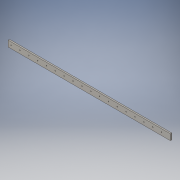
# Autodesk Inventor part: RailBar
Saved by Autodesk Inventor 2016 (Build 200138000, 138)
## iProperties
Created: 2015-08-23
Part Number: RailBar
Material: Stainless Steel
Document SubType Name: Modeling
Designer: myhome
Mass: 3520 g
Surface Area: 1108 cm^2
Volume: 440 cm^3
Density: 8 g/cm^3
Appearance: Semi-Polished
Author: myhome
Autodesk Inventor part; units mm, degrees
ref_plane "YZ Plane" through (0, 0, 0) normal (1, 0, 0) x (0, 1, 0)
ref_plane "XZ Plane" through (0, 0, 0) normal (0, 1, 0) x (-1, 0, 0)
ref_plane "XY Plane" through (0, 0, 0) normal (0, 0, 1) x (1, 0, 0)
sketch "Sketch1" plane through (0, 0, 0) normal (0, 0, 1) x (1, 0, 0)
  line L0 (0, 0) -> (1100, 0)
  line L1 (1100, 0) -> (1100, 40)
  line L2 (1100, 40) -> (0, 40)
  line L3 (0, 40) -> (0, 0)
  line L4 (1100, 40) -> (1040, 40)
  line L5 (1040, 40) -> (980, 40)
  line L6 (980, 40) -> (920, 40)
  line L7 (920, 40) -> (860, 40)
  line L8 (860, 40) -> (800, 40)
  line L9 (800, 40) -> (740, 40)
  line L10 (740, 40) -> (680, 40)
  line L11 (680, 40) -> (620, 40)
  line L12 (620, 40) -> (560, 40)
  line L13 (560, 40) -> (500, 40)
  line L14 (500, 40) -> (440, 40)
  line L15 (440, 40) -> (380, 40)
  line L16 (380, 40) -> (320, 40)
  line L17 (320, 40) -> (260, 40)
  line L18 (260, 40) -> (200, 40)
  line L19 (200, 40) -> (140, 40)
  line L20 (140, 40) -> (80, 40)
  line L21 (80, 40) -> (20, 40)
  circle A0 centre (1040, 20) radius 3
  circle A1 centre (980, 20) radius 3
  circle A2 centre (920, 20) radius 3
  circle A3 centre (860, 23) radius 3
  circle A4 centre (800, 20) radius 3
  circle A5 centre (740, 20) radius 3
  circle A6 centre (680, 20) radius 3
  circle A7 centre (560, 20) radius 3
  circle A8 centre (500, 20) radius 3
  circle A9 centre (440, 20) radius 3
  circle A10 centre (380, 20) radius 3
  circle A11 centre (320, 20) radius 3
  circle A12 centre (260, 20) radius 3
  circle A13 centre (200, 20) radius 3
  circle A14 centre (140, 20) radius 3
  circle A15 centre (80, 20) radius 3
  circle A16 centre (20, 20) radius 3
  dimension "d0" = 1100
  dimension "d1" = 40
  dimension "d22" = 6
  dimension "d23" = 6
  dimension "d24" = 6
  dimension "d25" = 6
  dimension "d26" = 6
  dimension "d27" = 6
  dimension "d28" = 6
  dimension "d30" = 6
  dimension "d31" = 6
  dimension "d32" = 6
  dimension "d33" = 6
  dimension "d34" = 6
  dimension "d35" = 6
  dimension "d36" = 6
  dimension "d38" = 6
  dimension "d39" = 6
  dimension "d40" = 6
  constraints: 42 end point, 17 centre point, 2 horizontal, 1 parallel, 1 perpendicular, 21 other
  measures "d0" distance of L1.end L3.start
  measures "d1" distance of L0.end L1.end
  measures "d22" diameter of A0
  measures "d23" diameter of A1
  measures "d24" diameter of A2
  measures "d25" diameter of A3
  measures "d26" diameter of A4
  measures "d27" diameter of A5
  measures "d28" diameter of A6
  measures "d30" diameter of A7
  measures "d31" diameter of A8
  measures "d32" diameter of A9
  measures "d33" diameter of A10
  measures "d34" diameter of A11
  measures "d35" diameter of A12
  measures "d36" diameter of A13
  measures "d38" diameter of A14
  measures "d39" diameter of A15
  measures "d40" diameter of A16
extrude "Extrusion1" add sketch "Sketch1" along normal blind 10 contours L3 L2 L1 L0 | A0 | A1 | A2 | A3 | A4 | A5 | A6 | A7 | A8 | A9 | A10 | A11 | A12 | A13 | A14 | A15 | A16
sketch "Sketch2" plane through (0, 0, 0) normal (0, 0, 1) x (1, 0, 0)
  line L0 (1100, 40) -> (0, 40) projected
  line L1 (0, 40) -> (0, 20)
  line L2 (0, 40) -> (0, 0) projected
  line L3 (1100, 20) -> (1040, 20)
  line L4 (1040, 20) -> (980, 20)
  line L5 (980, 20) -> (920, 20)
  line L6 (920, 20) -> (860, 20)
  line L7 (860, 20) -> (800, 20)
  line L8 (800, 20) -> (740, 20)
  line L9 (740, 20) -> (680, 20)
  line L10 (680, 20) -> (620, 20)
  line L11 (620, 20) -> (560, 20)
  line L12 (560, 20) -> (500, 20)
  line L13 (500, 20) -> (440, 20)
  line L14 (440, 20) -> (380, 20)
  line L15 (380, 20) -> (320, 20)
  line L16 (320, 20) -> (260, 20)
  line L17 (260, 20) -> (200, 20)
  line L18 (200, 20) -> (140, 20)
  line L19 (140, 20) -> (80, 20)
  line L20 (80, 20) -> (20, 20)
  circle A0 centre (740, 20) radius 3
  circle A1 centre (800, 20) radius 3
  circle A2 centre (860, 20) radius 3
  circle A3 centre (680, 20) radius 3
  circle A4 centre (1040, 20) radius 3
  circle A5 centre (980, 20) radius 3
  circle A6 centre (920, 20) radius 3
  circle A7 centre (620, 20) radius 3
  circle A8 centre (560, 20) radius 3
  circle A9 centre (500, 20) radius 3
  circle A10 centre (440, 20) radius 3
  circle A11 centre (380, 20) radius 3
  circle A12 centre (320, 20) radius 3
  circle A13 centre (260, 20) radius 3
  circle A14 centre (200, 20) radius 3
  circle A15 centre (140, 20) radius 3
  circle A16 centre (80, 20) radius 3
  circle A17 centre (20, 20) radius 3
  dimension "d41" = 60
  dimension "d42" = 60
  dimension "d43" = 60
  dimension "d44" = 60
  dimension "d45" = 60
  dimension "d46" = 60
  dimension "d47" = 60
  dimension "d48" = 60
  dimension "d49" = 60
  dimension "d50" = 60
  dimension "d51" = 60
  dimension "d52" = 60
  dimension "d53" = 60
  dimension "d54" = 60
  dimension "d55" = 60
  dimension "d56" = 60
  dimension "d57" = 60
  dimension "d58" = 60
  dimension "d59" = 6
  dimension "d60" = 6
  dimension "d61" = 6
  dimension "d62" = 6
  dimension "d63" = 6
  dimension "d64" = 6
  dimension "d65" = 6
  dimension "d66" = 6
  dimension "d67" = 6
  dimension "d68" = 6
  dimension "d69" = 6
  dimension "d70" = 6
  dimension "d71" = 6
  dimension "d72" = 6
  dimension "d73" = 6
  dimension "d74" = 6
  dimension "d75" = 6
  dimension "d76" = 6
  constraints: 38 end point, 18 centre point, 18 coincident, 17 point on line, 1 horizontal, 1 midpoint
  measures "d41" distance of L3.start L3.end
  measures "d42" distance of L3.end L4.end
  measures "d43" distance of L4.end L5.end
  measures "d44" distance of L5.end L6.end
  measures "d45" distance of L6.end L7.end
  measures "d46" distance of L7.end L8.end
  measures "d47" distance of L8.end L9.end
  measures "d48" distance of L9.end L10.end
  measures "d49" distance of L10.end L11.end
  measures "d50" distance of L11.end L12.end
  measures "d51" distance of L12.end L13.end
  measures "d52" distance of L13.end L14.end
  measures "d53" distance of L14.end L15.end
  measures "d54" distance of L15.end L16.end
  measures "d55" distance of L16.end L17.end
  measures "d56" distance of L17.end L18.end
  measures "d57" distance of L18.end L19.end
  measures "d58" distance of L19.end L20.end
  measures "d59" diameter of A0
  measures "d60" diameter of A1
  measures "d61" diameter of A2
  measures "d62" diameter of A3
  measures "d63" diameter of A4
  measures "d64" diameter of A5
  measures "d65" diameter of A6
  measures "d66" diameter of A7
  measures "d67" diameter of A8
  measures "d68" diameter of A9
  measures "d69" diameter of A10
  measures "d70" diameter of A11
  measures "d71" diameter of A12
  measures "d72" diameter of A13
  measures "d73" diameter of A14
  measures "d74" diameter of A15
  measures "d75" diameter of A16
  measures "d76" diameter of A17
extrude "Extrusion2" cut sketch "Sketch2" along normal mid plane 100
body "Solid1"
